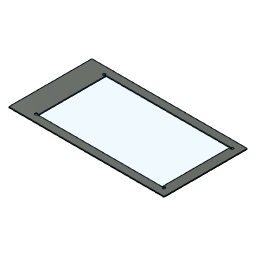
Power Supply Mounting Template (Autodesk Fusion 360 design; units mm, degrees)
Autodesk Fusion 360 part; units mm, degrees
sketch "Sketch1" plane through (0, 0, 0) normal (0, 0, 1) x (1, 0, 0)
  line L0 (88.5, -47.25) -> (-88.5, -47.25) construction
  line L1 (-88.5, -47.25) -> (-88.5, 47.25) construction
  line L2 (-88.5, 47.25) -> (88.5, 47.25) construction
  line L3 (88.5, 47.25) -> (88.5, -47.25) construction
  line L4 (88.5, -47.25) -> (-88.5, 47.25) construction
  line L5 (-88.5, -47.25) -> (88.5, 47.25) construction
  circle A0 centre (-88.5, 47.25) radius 1.75
  circle A1 centre (88.5, 47.25) radius 1.75
  circle A2 centre (88.5, -47.25) radius 1.75
  circle A3 centre (-88.5, -47.25) radius 1.75
  circle A4 centre (88.5, -47.25) radius 2.5
  circle A5 centre (88.5, 47.25) radius 2.5
  circle A6 centre (-88.5, 47.25) radius 2.5
  circle A7 centre (-88.5, -47.25) radius 2.5
  line L6 (86, -47.25) -> (-86, -47.25)
  line L7 (-86, -47.25) -> (-86, 47.25)
  line L8 (-86, 47.25) -> (86, 47.25)
  line L9 (86, 47.25) -> (86, -47.25)
  line L10 (86, -47.25) -> (-86, 47.25) construction
  line L11 (-86, -47.25) -> (86, 47.25) construction
  line L12 (99, -57.5) -> (-116, -57.5)
  line L13 (-116, -57.5) -> (-116, 57.5)
  line L14 (-116, 57.5) -> (99, 57.5)
  line L15 (99, 57.5) -> (99, -57.5)
  dimension "d1" = 177
  dimension "d2" = 94.5
  dimension "d3" = 3.5
  dimension "d4" = 3.5
  dimension "d5" = 3.5
  dimension "d6" = 3.5
  dimension "d7" = 5
  dimension "d8" = 5
  dimension "d9" = 5
  dimension "d10" = 5
  dimension "d11" = 215
  dimension "d12" = 115
  dimension "d15" = 27.5
  dimension "d16" = 57.5
  constraint horizontal L0
  constraint perpendicular L0 L1
  constraint parallel L0 L2
  constraint parallel L1 L3
  constraint coincident L4 origin
  constraint coincident L5 origin
  constraint coincident L1.end L2.start
  constraint coincident L2.end L3.start
  constraint coincident L0.start L3.end
  constraint coincident L0.end L1.start
  constraint concentric A2 A4
  constraint concentric A1 A5
  constraint concentric A0 A6
  constraint concentric A3 A7
  constraint horizontal L6
  constraint perpendicular L6 L7
  constraint parallel L6 L8
  constraint parallel L7 L9
  constraint coincident L0 L6.start
  constraint coincident A4 L6.start
  constraint coincident L10 origin
  constraint coincident L11 origin
  constraint horizontal L12
  constraint perpendicular L12 L13
  constraint parallel L12 L14
  constraint parallel L13 L15
  measures "d1" distance of L1.end L2.end
  measures "d2" distance of L0.end L1.end
  measures "d3" diameter of A0
  measures "d4" diameter of A1
  measures "d5" diameter of A2
  measures "d6" diameter of A3
  measures "d7" diameter of A4
  measures "d8" diameter of A5
  measures "d9" diameter of A6
  measures "d10" diameter of A7
  measures "d11" distance of L13.end L14.end
  measures "d12" distance of L12.end L13.end
  measures "d15" distance of L1.end L13
  measures "d16" distance of L14 origin
extrude "Extrude1" add sketch "Sketch1" along normal blind 1 contours A4 | A7 | A6 | A5 | L12 L13 L14 L15
sketch "Sketch2" plane through (0, 0, 1) normal (0, 0, 1) x (-1, 0, 0)
  circle A0 centre (-88.5, -47.25) radius 1.75
  circle A1 centre (88.5, -47.25) radius 1.75
  line L0 (86, -47.25) -> (-86, -47.25)
  line L1 (-86, -47.25) -> (-86, 47.25)
  line L2 (-86, 47.25) -> (86, 47.25)
  line L3 (86, 47.25) -> (86, -47.25)
  circle A2 centre (88.5, 47.25) radius 1.75
  circle A3 centre (-88.5, 47.25) radius 1.75
  line L4 (-99, -57.5) -> (116, -57.5)
  line L5 (116, -57.5) -> (116, 57.5)
  line L6 (116, 57.5) -> (-99, 57.5)
  line L7 (-99, 57.5) -> (-99, -57.5)
